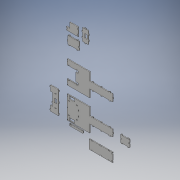
# Autodesk Inventor part: Radio Dowser
Saved by Autodesk Inventor 2018 (Build 220112000, 112)
## iProperties
Created: 2019-04-05
Part Number: Radio Dowser
Material: Generic
Document SubType Name: Modeling
Designer: rpoulter
Density: 1 g/cm^3
Appearance: Default
Author: rpoulter
Autodesk Inventor part; units mm, degrees
ref_plane "YZ Plane" through (0, 0, 0) normal (1, 0, 0) x (0, 1, 0)
ref_plane "XZ Plane" through (0, 0, 0) normal (0, 1, 0) x (-1, 0, 0)
ref_plane "XY Plane" through (0, 0, 0) normal (0, 0, 1) x (1, 0, 0)
sketch "microbit platform" plane through (0, 0, 0) normal (0, 1, 0) x (-1, 0, 0)
  line L0 (0, 0) -> (-46, 0)
  line L1 (-46, 0) -> (-46, -53)
  line L2 (-46, -53) -> (0, -53)
  line L3 (0, -53) -> (0, 0)
  line L4 (-46, -12.5) -> (-43, -12.5)
  line L5 (-43, -12.5) -> (-43, -17.5)
  line L6 (-43, -17.5) -> (-46, -17.5)
  line L7 (-46, -17.5) -> (-46, -12.5)
  line L8 (-46, -35.5) -> (-43, -35.5)
  line L9 (-43, -35.5) -> (-43, -40.5)
  line L10 (-43, -40.5) -> (-46, -40.5)
  line L11 (-46, -40.5) -> (-46, -35.5)
  line L12 (-46, -53) -> (0, -53)
  line L13 (0, -53) -> (0, -45)
  line L14 (0, -45) -> (-46, -45)
  line L15 (-46, -45) -> (-46, -53)
  line L16 (-46, 0) -> (0, 0)
  line L17 (0, 0) -> (0, -8)
  line L18 (0, -8) -> (-46, -8)
  line L19 (-46, -8) -> (-46, 0)
  line L20 (0, 0) -> (-9, 0)
  line L21 (-9, 0) -> (-9, -31)
  line L22 (-9, -31) -> (0, -31)
  line L23 (0, -31) -> (0, 0)
  line L24 (0, -31) -> (6, -31)
  line L25 (6, -31) -> (6, -35.5)
  line L26 (6, -35.5) -> (0, -35.5)
  line L27 (0, -35.5) -> (0, -31)
  line L28 (0, -40.5) -> (6, -40.5)
  line L29 (6, -40.5) -> (6, -45)
  line L30 (6, -45) -> (0, -45)
  line L31 (0, -45) -> (0, -40.5)
  line L32 (0, -40.5) -> (3, -40.5)
  line L33 (3, -40.5) -> (3, -35.5)
  line L34 (3, -35.5) -> (0, -35.5)
  line L35 (0, -35.5) -> (0, -40.5)
  point P0 (0, -35.5)
  dimension "d17" = 46
  dimension "d18" = 53
  dimension "d21" = 3
  dimension "d22" = 5
  dimension "d23" = 5
  dimension "d24" = 8
  dimension "d25" = 8
  dimension "d26" = 9
  dimension "d27" = 31
  dimension "d29" = 4.5
  dimension "d140" = 6
  dimension "d226" = 3
  constraints: 72 end point, 18 parallel, 9 horizontal, 9 perpendicular, 7 point on line, 1 midpoint
  measures "d17" distance of L2.end L1.end
  measures "d18" distance of L1.end L0.end
  measures "d21" distance of L5.end L6.end
  measures "d22" distance of L4.end L5.end
  measures "d23" distance of L8.end L9.end
  measures "d24" distance of L13.end L12.end
  measures "d25" distance of L16.end L17.end
  measures "d26" distance of L22.end L21.end
  measures "d27" distance of L21.end L20.end
  measures "d29" distance between parallel lines of L18 L4
  measures "d140" distance of L25.end L26.end
  measures "d226" distance of L34.end L33.end
extrude "microbit bed" add sketch "microbit platform" along normal blind 3 contours L21 L22 L3 L14 L1 L10 L9 L8 L6 L5 L4 L18 | L24 L25 L26 L3 | L26 L33 L28 L3 | L28 L29 L30 L3
sketch "bed support bottom" plane through (0, 0, 0) normal (0, 1, 0) x (-1, 0, 0)
  line L0 (-46, -8) -> (-46, -12.5) projected
  line L1 (-65.1607, -0.0001) -> (-65.1607, -12.5001)
  line L2 (-46, -12.5) -> (-43, -12.5) projected
  line L3 (-65.1607, -12.5001) -> (-62.1607, -12.5001)
  line L4 (-43, -12.5) -> (-43, -17.5) projected
  line L5 (-62.1607, -12.5001) -> (-62.1607, -17.5001)
  line L6 (-43, -17.5) -> (-46, -17.5) projected
  line L7 (-62.1607, -17.5001) -> (-65.0584, -17.5001)
  line L8 (-46, -17.5) -> (-46, -35.5) projected
  line L9 (-65.0584, -17.5001) -> (-65.0584, -35.5001)
  line L10 (-43, -35.5) -> (-46, -35.5) projected
  line L11 (-65.0584, -35.5001) -> (-62.1607, -35.5001)
  line L12 (-43, -35.5) -> (-43, -40.5) projected
  line L13 (-62.1607, -35.5001) -> (-62.1607, -40.5001)
  line L14 (-43, -40.5) -> (-46, -40.5) projected
  line L15 (-62.1607, -40.5001) -> (-65.0584, -40.5001)
  line L16 (-65.0584, -40.5001) -> (-65.0584, -53.0001)
  line L17 (-90.0584, -53.0001) -> (-90.0584, -40.5001)
  line L18 (-90.0584, -40.5001) -> (-93.0584, -40.5001)
  line L19 (-93.0584, -40.5001) -> (-93.0584, -35.5001)
  line L20 (-93.0584, -35.5001) -> (-90.0584, -35.5001)
  line L21 (-90.0584, -17.5001) -> (-93.0584, -17.5001)
  line L22 (-93.0584, -12.5001) -> (-90.0584, -12.5001)
  line L23 (-90.0584, -17.5001) -> (-90.0584, -35.5001)
  line L24 (-93.0584, -17.5001) -> (-93.0584, -12.5001)
  line L25 (-90.0584, -0.0001) -> (-90.0584, -12.5001)
  line L26 (-80.0584, -0.0001) -> (-80.0584, 2.9999)
  line L27 (-80.0584, 2.9999) -> (-75.0584, 2.9999)
  line L28 (-75.0584, 2.9999) -> (-75.0584, -0.0001)
  line L29 (-80.0584, -53.0001) -> (-80.0584, -56.0001)
  line L30 (-80.0584, -56.0001) -> (-75.0584, -56.0001)
  line L31 (-75.0584, -56.0001) -> (-75.0584, -53.0001)
  line L32 (-65.1607, -0.0001) -> (-75.0584, -0.0001)
  line L33 (-80.0584, -0.0001) -> (-90.0584, -0.0001)
  line L34 (-65.0584, -53.0001) -> (-75.0584, -53.0001)
  line L35 (-80.0584, -53.0001) -> (-90.0584, -53.0001)
  line L36 (-75.0584, -17.5001) -> (-85.0584, -17.5001)
  line L37 (-85.0584, -17.5001) -> (-85.0584, -35.5001)
  line L38 (-85.0584, -35.5001) -> (-75.0584, -35.5001)
  line L39 (-75.0584, -35.5001) -> (-75.0584, -17.5001)
  point P0 (0, 0)
  dimension "d32" = 25
  dimension "d33" = 3
  dimension "d49" = 10
  dimension "d146" = 10
  dimension "d220" = 5
  dimension "d221" = 17.5
  constraints: 64 end point, 14 point on line, 12 parallel, 7 perpendicular, 3 horizontal, 2 vertical
  measures "d32" distance of L16.end L17.start
  measures "d33" distance of L17.end L18.end
  measures "d49" distance between parallel lines of L25 L26
  measures "d146" distance between parallel lines of L37 L39
  measures "d220" distance between parallel lines of L23 L37
  measures "d221" distance between parallel lines of L35 L38
sketch "bed support side x2" plane through (0, 0, 0) normal (0, 1, 0) x (-1, 0, 0)
  line L0 (-46.5564, -81.0331) -> (-43.5564, -81.0331)
  line L1 (-43.5564, -81.0331) -> (-43.5564, -86.0331)
  line L2 (-43.5564, -86.0331) -> (-46.5564, -86.0331)
  line L3 (-8.5564, -96.0331) -> (-8.5564, -99.0331)
  line L4 (-8.5564, -99.0331) -> (-3.5564, -99.0331)
  line L5 (-3.5564, -99.0331) -> (-3.5564, -96.0331)
  line L6 (-38.5564, -96.0331) -> (-38.5564, -99.0331)
  line L7 (-38.5564, -99.0331) -> (-43.5564, -99.0331)
  line L8 (-43.5564, -99.0331) -> (-43.5564, -96.0331)
  line L9 (-46.5564, -71.0331) -> (-46.5564, -62.0331)
  line L10 (-0.5564, -62.0331) -> (-0.5564, -71.0331)
  line L11 (-8.5564, -62.0331) -> (-8.5564, -59.0331)
  line L12 (-8.5564, -59.0331) -> (-3.5564, -59.0331)
  line L13 (-3.5564, -59.0331) -> (-3.5564, -62.0331)
  line L14 (-38.5564, -62.0331) -> (-38.5564, -59.0331)
  line L15 (-38.5564, -59.0331) -> (-43.5564, -59.0331)
  line L16 (-43.5564, -59.0331) -> (-43.5564, -62.0331)
  line L17 (-3.5564, -62.0331) -> (-0.5564, -62.0331)
  line L18 (-46.5564, -62.0331) -> (-43.5564, -62.0331)
  line L19 (-38.5564, -62.0331) -> (-8.5564, -62.0331)
  line L20 (-3.5564, -96.0331) -> (-0.5564, -96.0331)
  line L21 (-46.5564, -96.0331) -> (-43.5564, -96.0331)
  line L22 (-38.5564, -96.0331) -> (-8.5564, -96.0331)
  line L23 (-46.5564, -71.0331) -> (-46.5564, -81.0331)
  line L24 (-46.5564, -86.0331) -> (-46.5564, -96.0331)
  line L25 (-0.5564, -96.0331) -> (-0.5564, -86.0331)
  line L26 (-0.5564, -81.0331) -> (-0.5564, -71.0331)
  line L27 (-0.5564, -81.0331) -> (2.4436, -81.0331)
  line L28 (2.4436, -81.0331) -> (2.4436, -86.0331)
  line L29 (2.4436, -86.0331) -> (-0.5564, -86.0331)
  line L30 (-46.5564, -96.0331) -> (-49.5564, -96.0331)
  line L31 (-49.5564, -96.0331) -> (-49.5564, -86.0331)
  line L32 (-49.5564, -86.0331) -> (-46.5564, -86.0331)
  line L33 (-46.5564, -81.0331) -> (-49.5564, -81.0331)
  line L34 (-49.5564, -81.0331) -> (-49.5564, -62.0331)
  line L35 (-49.5564, -62.0331) -> (-46.5564, -62.0331)
  line L36 (-46.5564, -86.0331) -> (-46.5564, -81.0331)
  point P0 (0, 0)
  dimension "d227" = 3
  dimension "d228" = 3
  constraints: 74 end point, 11 parallel, 9 perpendicular, 9 point on line, 3 collinear, 3 horizontal
  measures "d227" distance of L21.start L8.end
  measures "d228" distance of L21.start L30.end
sketch "top plate" plane through (0, 0, 0) normal (0, 1, 0) x (-1, 0, 0)
  line L0 (3, -153.8907) -> (-97, -153.8907)
  line L1 (-97, -153.8907) -> (-97, -253.8907)
  line L2 (-97, -253.8907) -> (3, -253.8907)
  line L3 (3, -253.8907) -> (3, -153.8907)
  line L4 (3, -177.3907) -> (-46, -177.3907)
  line L5 (-46, -177.3907) -> (-46, -230.3907)
  line L6 (-46, -230.3907) -> (3, -230.3907)
  line L7 (3, -230.3907) -> (3, -177.3907)
  line L8 (-46, -185.3907) -> (-36, -185.3907)
  line L9 (-36, -185.3907) -> (-36, -222.3907)
  line L10 (-36, -222.3907) -> (-46, -222.3907)
  line L11 (-46, -222.3907) -> (-46, -185.3907)
  line L12 (3, -156.595) -> (0, -156.595)
  line L13 (0, -156.595) -> (0, -161.595)
  line L14 (0, -161.595) -> (3, -161.595)
  line L15 (3, -161.595) -> (3, -156.595)
  line L16 (3, -251.316) -> (0, -251.316)
  line L17 (0, -251.316) -> (0, -246.316)
  line L18 (0, -246.316) -> (3, -246.316)
  line L19 (3, -246.316) -> (3, -251.316)
  line L20 (-43, -177.3907) -> (-38, -177.3907)
  line L21 (-38, -177.3907) -> (-38, -174.3907)
  line L22 (-38, -174.3907) -> (-43, -174.3907)
  line L23 (-43, -174.3907) -> (-43, -177.3907)
  line L24 (-8, -177.3907) -> (-3, -177.3907)
  line L25 (-3, -177.3907) -> (-3, -174.3907)
  line L26 (-3, -174.3907) -> (-8, -174.3907)
  line L27 (-8, -174.3907) -> (-8, -177.3907)
  line L28 (-43, -230.3907) -> (-38, -230.3907)
  line L29 (-38, -230.3907) -> (-38, -233.3907)
  line L30 (-38, -233.3907) -> (-43, -233.3907)
  line L31 (-43, -233.3907) -> (-43, -230.3907)
  line L32 (-3, -230.3907) -> (-8, -230.3907)
  line L33 (-8, -230.3907) -> (-8, -233.3907)
  line L34 (-8, -233.3907) -> (-3, -233.3907)
  line L35 (-3, -233.3907) -> (-3, -230.3907)
  line L36 (-97, -188.8907) -> (-197, -188.8907)
  line L37 (-197, -188.8907) -> (-197, -218.8907)
  line L38 (-197, -218.8907) -> (-97, -218.8907)
  line L39 (-97, -218.8907) -> (-97, -188.8907)
  line L40 (-107, -218.8907) -> (-112, -218.8907)
  line L41 (-112, -218.8907) -> (-112, -221.8907)
  line L42 (-112, -221.8907) -> (-107, -221.8907)
  line L43 (-107, -221.8907) -> (-107, -218.8907)
  line L44 (-107, -188.8907) -> (-112, -188.8907)
  line L45 (-112, -188.8907) -> (-112, -185.8907)
  line L46 (-112, -185.8907) -> (-107, -185.8907)
  line L47 (-107, -185.8907) -> (-107, -188.8907)
  line L48 (-144.5, -218.8907) -> (-149.5, -218.8907)
  line L49 (-149.5, -218.8907) -> (-149.5, -221.8907)
  line L50 (-149.5, -221.8907) -> (-144.5, -221.8907)
  line L51 (-144.5, -221.8907) -> (-144.5, -218.8907)
  line L52 (-144.5, -188.8907) -> (-149.5, -188.8907)
  line L53 (-149.5, -188.8907) -> (-149.5, -185.8907)
  line L54 (-149.5, -185.8907) -> (-144.5, -185.8907)
  line L55 (-144.5, -185.8907) -> (-144.5, -188.8907)
  line L56 (-182, -218.8907) -> (-187, -218.8907)
  line L57 (-187, -218.8907) -> (-187, -221.8907)
  line L58 (-187, -221.8907) -> (-182, -221.8907)
  line L59 (-182, -221.8907) -> (-182, -218.8907)
  line L60 (-182, -188.8907) -> (-187, -188.8907)
  line L61 (-187, -188.8907) -> (-187, -185.8907)
  line L62 (-187, -185.8907) -> (-182, -185.8907)
  line L63 (-182, -185.8907) -> (-182, -188.8907)
  line L64 (-197, -201.3907) -> (-200, -201.3907)
  line L65 (-200, -201.3907) -> (-200, -206.3907)
  line L66 (-200, -206.3907) -> (-197, -206.3907)
  line L67 (-197, -206.3907) -> (-197, -201.3907)
  point P0 (0, 0)
  dimension "d63" = 100
  dimension "d64" = 100
  dimension "d65" = 49
  dimension "d66" = 53
  dimension "d67" = 23.5
  dimension "d68" = 10
  dimension "d69" = 37
  dimension "d70" = 8
  dimension "d71" = 3
  dimension "d72" = 5
  dimension "d73" = 3
  dimension "d74" = 5
  dimension "d75" = 5
  dimension "d76" = 3
  dimension "d77" = 3
  dimension "d78" = 5
  dimension "d79" = 3
  dimension "d80" = 30
  dimension "d81" = 3
  dimension "d162" = 100
  dimension "d163" = 30
  dimension "d164" = 35
  dimension "d165" = 5
  dimension "d166" = 3
  dimension "d167" = 3
  dimension "d168" = 5
  dimension "d169" = 5
  dimension "d170" = 3
  dimension "d171" = 5
  dimension "d172" = 12.5
  dimension "d173" = 10
  dimension "d174" = 10
  dimension "d175" = 47.5
  constraints: 136 end point, 34 parallel, 22 point on line, 17 horizontal, 17 perpendicular, 2 collinear
  measures "d63" distance of L2.end L1.end
  measures "d64" distance of L1.end L0.end
  measures "d65" distance of L6.end L5.end
  measures "d66" distance of L5.end L4.end
  measures "d67" distance between parallel lines of L0 L4
  measures "d68" distance of L9.end L10.end
  measures "d69" distance of L8.end L9.end
  measures "d70" distance between parallel lines of L4 L8
  measures "d71" distance of L14.end L13.end
  measures "d72" distance of L13.end L12.end
  measures "d73" distance of L17.end L18.end
  measures "d74" distance of L16.end L17.end
  measures "d75" distance of L22.end L21.end
  measures "d76" distance of L21.end L20.end
  measures "d77" distance between parallel lines of L5 L23
  measures "d78" distance of L26.end L25.end
  measures "d79" distance of L25.end L24.end
  measures "d80" distance between parallel lines of L27 L21
  measures "d81" distance of L28.end L29.end
  measures "d162" distance of L38.end L37.end
  measures "d163" distance of L37.end L36.end
  measures "d164" distance between parallel lines of L0 L36
  measures "d165" distance of L42.end L41.end
  measures "d166" distance of L41.end L40.end
  measures "d167" distance of L44.end L45.end
  measures "d168" distance of L50.end L49.end
  measures "d169" distance of L58.end L57.end
  measures "d170" distance of L66.end L65.end
  measures "d171" distance of L65.end L64.end
  measures "d172" distance between parallel lines of L36 L64
  measures "d173" distance between parallel lines of L37 L57
  measures "d174" distance between parallel lines of L1 L43
  measures "d175" distance between parallel lines of L37 L49
sketch "bottom plate" plane through (0, 0, 0) normal (0, 1, 0) x (-1, 0, 0)
  line L0 (3, -288.3381) -> (-97, -288.3381)
  line L1 (-97, -288.3381) -> (-97, -388.3381)
  line L2 (-97, -388.3381) -> (3, -388.3381)
  line L3 (3, -388.3381) -> (3, -288.3381)
  line L4 (3, -364.8381) -> (3, -311.8381)
  line L5 (3, -291.0423) -> (0, -291.0423)
  line L6 (0, -291.0423) -> (0, -296.0423)
  line L7 (0, -296.0423) -> (3, -296.0423)
  line L8 (3, -296.0423) -> (3, -291.0423)
  line L9 (3, -385.7634) -> (0, -385.7634)
  line L10 (0, -385.7634) -> (0, -380.7634)
  line L11 (0, -380.7634) -> (3, -380.7634)
  line L12 (3, -380.7634) -> (3, -385.7634)
  line L13 (-43, -311.8381) -> (-38, -311.8381)
  line L14 (-38, -311.8381) -> (-38, -308.8381)
  line L15 (-38, -308.8381) -> (-43, -308.8381)
  line L16 (-43, -308.8381) -> (-43, -311.8381)
  line L17 (-8, -311.8381) -> (-3, -311.8381)
  line L18 (-3, -311.8381) -> (-3, -308.8381)
  line L19 (-3, -308.8381) -> (-8, -308.8381)
  line L20 (-8, -308.8381) -> (-8, -311.8381)
  line L21 (-43, -364.8381) -> (-38, -364.8381)
  line L22 (-38, -364.8381) -> (-38, -367.8381)
  line L23 (-38, -367.8381) -> (-43, -367.8381)
  line L24 (-43, -367.8381) -> (-43, -364.8381)
  line L25 (-3, -364.8381) -> (-8, -364.8381)
  line L26 (-8, -364.8381) -> (-8, -367.8381)
  line L27 (-8, -367.8381) -> (-3, -367.8381)
  line L28 (-3, -367.8381) -> (-3, -364.8381)
  line L29 (-46, -324.3381) -> (-49, -324.3381)
  line L30 (-49, -324.3381) -> (-49, -329.3381)
  line L31 (-49, -329.3381) -> (-46, -329.3381)
  line L32 (-46, -329.3381) -> (-46, -324.3381)
  line L33 (-46, -352.3381) -> (-49, -352.3381)
  line L34 (-49, -352.3381) -> (-49, -347.3381)
  line L35 (-49, -347.3381) -> (-46, -347.3381)
  line L36 (-46, -347.3381) -> (-46, -352.3381)
  line L37 (-7, -373.3381) -> (-29, -373.3381)
  line L38 (-29, -373.3381) -> (-29, -385.3381)
  line L39 (-29, -385.3381) -> (-7, -385.3381)
  line L40 (-7, -385.3381) -> (-7, -373.3381)
  line L41 (-7, -291.3381) -> (-29, -291.3381)
  line L42 (-29, -291.3381) -> (-29, -303.3381)
  line L43 (-29, -303.3381) -> (-7, -303.3381)
  line L44 (-7, -303.3381) -> (-7, -291.3381)
  line L45 (3, -335.8381) -> (0, -335.8381)
  line L46 (0, -335.8381) -> (0, -340.8381)
  line L47 (0, -340.8381) -> (3, -340.8381)
  line L48 (3, -340.8381) -> (3, -335.8381)
  line L49 (-97, -323.3381) -> (-197, -323.3381)
  line L50 (-197, -323.3381) -> (-197, -353.3381)
  line L51 (-197, -353.3381) -> (-97, -353.3381)
  line L52 (-97, -353.3381) -> (-97, -323.3381)
  line L53 (-197, -335.8381) -> (-200, -335.8381)
  line L54 (-200, -335.8381) -> (-200, -340.8381)
  line L55 (-200, -340.8381) -> (-197, -340.8381)
  line L56 (-197, -340.8381) -> (-197, -335.8381)
  line L57 (-107, -323.3381) -> (-112, -323.3381)
  line L58 (-112, -323.3381) -> (-112, -320.3381)
  line L59 (-112, -320.3381) -> (-107, -320.3381)
  line L60 (-107, -320.3381) -> (-107, -323.3381)
  line L61 (-187, -323.3381) -> (-182, -323.3381)
  line L62 (-182, -323.3381) -> (-182, -320.3381)
  line L63 (-182, -320.3381) -> (-187, -320.3381)
  line L64 (-187, -320.3381) -> (-187, -323.3381)
  line L65 (-144.5, -323.3381) -> (-149.5, -323.3381)
  line L66 (-149.5, -323.3381) -> (-149.5, -320.3381)
  line L67 (-149.5, -320.3381) -> (-144.5, -320.3381)
  line L68 (-144.5, -320.3381) -> (-144.5, -323.3381)
  line L69 (-107, -353.3381) -> (-112, -353.3381)
  line L70 (-112, -353.3381) -> (-112, -356.3381)
  line L71 (-112, -356.3381) -> (-107, -356.3381)
  line L72 (-107, -356.3381) -> (-107, -353.3381)
  line L73 (-182, -353.3381) -> (-187, -353.3381)
  line L74 (-187, -353.3381) -> (-187, -356.3381)
  line L75 (-187, -356.3381) -> (-182, -356.3381)
  line L76 (-182, -356.3381) -> (-182, -353.3381)
  line L77 (-144.5, -353.3381) -> (-149.5, -353.3381)
  line L78 (-149.5, -353.3381) -> (-149.5, -356.3381)
  line L79 (-149.5, -356.3381) -> (-144.5, -356.3381)
  line L80 (-144.5, -356.3381) -> (-144.5, -353.3381)
  point P0 (0, 0)
  dimension "d82" = 100
  dimension "d83" = 100
  dimension "d90" = 3
  dimension "d91" = 5
  dimension "d92" = 3
  dimension "d93" = 5
  dimension "d94" = 5
  dimension "d95" = 3
  dimension "d97" = 5
  dimension "d98" = 3
  dimension "d99" = 30
  dimension "d100" = 3
  dimension "d101" = 3
  dimension "d102" = 5
  dimension "d103" = 5
  dimension "d104" = 20.5
  dimension "d105" = 12.5
  dimension "d106" = 20.5
  dimension "d108" = 12.5
  dimension "d113" = 22
  dimension "d114" = 12
  dimension "d115" = 3
  dimension "d116" = 10
  dimension "d117" = 22
  dimension "d118" = 12
  dimension "d119" = 5
  dimension "d120" = 47.5
  dimension "d150" = 100
  dimension "d151" = 30
  dimension "d152" = 35
  dimension "d153" = 3
  dimension "d154" = 5
  dimension "d155" = 3
  dimension "d156" = 5
  dimension "d157" = 5
  dimension "d158" = 3
  dimension "d159" = 10
  dimension "d160" = 10
  dimension "d161" = 47.5
  dimension "d213" = 3
  constraints: 162 end point, 40 parallel, 23 point on line, 20 horizontal, 20 perpendicular
  measures "d82" distance of L2.end L2.start
  measures "d83" distance of L2.start L0.end
  measures "d90" distance of L7.end L7.start
  measures "d91" distance of L7.start L5.end
  measures "d92" distance of L10.end L11.end
  measures "d93" distance of L9.end L10.end
  measures "d94" distance of L16.start L14.end
  measures "d95" distance of L14.end L14.start
  measures "d97" distance of L20.start L18.end
  measures "d98" distance of L18.end L18.start
  measures "d99" distance between parallel lines of L20 L14
  measures "d100" distance of L21.end L23.start
  measures "d101" distance of L31.end L30.end
  measures "d102" distance of L30.end L29.end
  measures "d103" distance of L33.end L34.end
  measures "d104" distance between parallel lines of L0 L15
  measures "d105" distance between parallel lines of L13 L29
  measures "d106" distance between parallel lines of L2 L23
  measures "d108" distance between parallel lines of L21 L33
  measures "d113" distance of L39.end L38.end
  measures "d114" distance of L38.end L37.end
  measures "d115" distance between parallel lines of L2 L39
  measures "d116" distance between parallel lines of L3 L40
  measures "d117" distance of L43.end L42.end
  measures "d118" distance of L42.end L41.end
  measures "d119" distance of L46.end L45.end
  measures "d120" distance between parallel lines of L0 L45
  measures "d150" distance of L51.end L50.end
  measures "d151" distance of L50.end L49.end
  measures "d152" distance between parallel lines of L0 L49
  measures "d153" distance of L55.end L54.end
  measures "d154" distance of L58.end L59.end
  measures "d155" distance of L57.end L58.end
  measures "d156" distance of L63.end L62.end
  measures "d157" distance of L66.end L67.end
  measures "d158" distance of L70.end L69.end
  measures "d159" distance between parallel lines of L1 L60
  measures "d160" distance between parallel lines of L50 L64
  measures "d161" distance between parallel lines of L50 L66
  measures "d213" distance between parallel lines of L0 L41
sketch "side support top" plane through (0, 0, 0) normal (0, 1, 0) x (-1, 0, 0)
  line L0 (42.0704, -291.2579) -> (76.0704, -291.2579)
  line L1 (76.0704, -291.2579) -> (76.0704, -391.2579)
  line L2 (76.0704, -391.2579) -> (42.0704, -391.2579)
  line L3 (42.0704, -391.2579) -> (42.0704, -291.2579)
  line L4 (42.0704, -294.2579) -> (39.0704, -294.2579)
  line L5 (39.0704, -294.2579) -> (39.0704, -299.2579)
  line L6 (39.0704, -299.2579) -> (42.0704, -299.2579)
  line L7 (42.0704, -299.2579) -> (42.0704, -294.2579)
  line L8 (42.0704, -388.2579) -> (39.0704, -388.2579)
  line L9 (39.0704, -388.2579) -> (39.0704, -383.2579)
  line L10 (39.0704, -383.2579) -> (42.0704, -383.2579)
  line L11 (42.0704, -383.2579) -> (42.0704, -388.2579)
  line L12 (42.0704, -338.7579) -> (39.0704, -338.7579)
  line L13 (39.0704, -338.7579) -> (39.0704, -343.7579)
  line L14 (39.0704, -343.7579) -> (42.0704, -343.7579)
  line L15 (42.0704, -343.7579) -> (42.0704, -338.7579)
  line L16 (76.0704, -294.2579) -> (79.0704, -294.2579)
  line L17 (79.0704, -294.2579) -> (79.0704, -299.2579)
  line L18 (79.0704, -299.2579) -> (76.0704, -299.2579)
  line L19 (76.0704, -299.2579) -> (76.0704, -294.2579)
  line L20 (76.0704, -388.2579) -> (79.0704, -388.2579)
  line L21 (79.0704, -388.2579) -> (79.0704, -383.2579)
  line L22 (79.0704, -383.2579) -> (76.0704, -383.2579)
  line L23 (76.0704, -383.2579) -> (76.0704, -388.2579)
  line L24 (76.0704, -314.7579) -> (67.0704, -314.7579)
  line L25 (67.0704, -314.7579) -> (67.0704, -367.7579)
  line L26 (67.0704, -367.7579) -> (76.0704, -367.7579)
  line L27 (76.0704, -367.7579) -> (76.0704, -314.7579)
  line L28 (57.0704, -367.7579) -> (52.0704, -367.7579)
  line L29 (52.0704, -367.7579) -> (52.0704, -370.7579)
  line L30 (52.0704, -370.7579) -> (57.0704, -370.7579)
  line L31 (57.0704, -370.7579) -> (57.0704, -367.7579)
  line L32 (57.0704, -314.7579) -> (52.0704, -314.7579)
  line L33 (52.0704, -314.7579) -> (52.0704, -311.7579)
  line L34 (52.0704, -311.7579) -> (57.0704, -311.7579)
  line L35 (57.0704, -311.7579) -> (57.0704, -314.7579)
  line L36 (59.0704, -332.2579) -> (49.0704, -332.2579)
  line L37 (49.0704, -332.2579) -> (49.0704, -350.2579)
  line L38 (49.0704, -350.2579) -> (59.0704, -350.2579)
  line L39 (59.0704, -350.2579) -> (59.0704, -332.2579)
  line L40 (67.0704, -355.2579) -> (70.0704, -355.2579)
  line L41 (70.0704, -355.2579) -> (70.0704, -350.2579)
  line L42 (70.0704, -350.2579) -> (67.0704, -350.2579)
  point P0 (0, 0)
  dimension "d121" = 34
  dimension "d122" = 100
  dimension "d123" = 3
  dimension "d124" = 5
  dimension "d125" = 5
  dimension "d126" = 5
  dimension "d127" = 3
  dimension "d128" = 5
  dimension "d129" = 3
  dimension "d130" = 3
  dimension "d131" = 47.5
  dimension "d132" = 9
  dimension "d133" = 53
  dimension "d134" = 23.5
  dimension "d142" = 5
  dimension "d143" = 3
  dimension "d144" = 10
  dimension "d145" = 3
  dimension "d147" = 10
  dimension "d148" = 18
  dimension "d149" = 41
  dimension "d224" = 3
  dimension "d225" = 5
  constraints: 86 end point, 21 parallel, 14 point on line, 11 horizontal, 11 perpendicular
  measures "d121" distance of L1.end L2.end
  measures "d122" distance of L0.end L1.end
  measures "d123" distance of L6.end L5.end
  measures "d124" distance of L5.end L4.end
  measures "d125" distance of L8.end L9.end
  measures "d126" distance of L13.end L12.end
  measures "d127" distance of L17.end L18.end
  measures "d128" distance of L16.end L17.end
  measures "d129" distance between parallel lines of L0 L4
  measures "d130" distance between parallel lines of L2 L8
  measures "d131" distance between parallel lines of L0 L12
  measures "d132" distance of L26.end L25.end
  measures "d133" distance of L25.end L24.end
  measures "d134" distance between parallel lines of L0 L24
  measures "d142" distance of L30.end L29.end
  measures "d143" distance of L29.end L28.end
  measures "d144" distance between parallel lines of L29 L3
  measures "d145" distance of L32.end L33.end
  measures "d147" distance of L38.end L37.end
  measures "d148" distance of L37.end L36.end
  measures "d149" distance between parallel lines of L0 L36
  measures "d224" distance of L42.end L41.end
  measures "d225" distance of L41.end L40.end
sketch "battery side" plane through (0, 0, 0) normal (0, 1, 0) x (-1, 0, 0)
  line L0 (-94.5331, -411.6252) -> (-197.5331, -411.6252)
  line L1 (-197.5331, -411.6252) -> (-197.5331, -451.6252)
  line L2 (-197.5331, -451.6252) -> (-94.5331, -451.6252)
  line L3 (-94.5331, -451.6252) -> (-94.5331, -411.6252)
  line L4 (-104.5331, -411.6252) -> (-109.5331, -411.6252)
  line L5 (-109.5331, -411.6252) -> (-109.5331, -414.6252)
  line L6 (-109.5331, -414.6252) -> (-104.5331, -414.6252)
  line L7 (-104.5331, -414.6252) -> (-104.5331, -411.6252)
  line L8 (-104.5331, -451.6252) -> (-109.5331, -451.6252)
  line L9 (-109.5331, -451.6252) -> (-109.5331, -448.6252)
  line L10 (-109.5331, -448.6252) -> (-104.5331, -448.6252)
  line L11 (-104.5331, -448.6252) -> (-104.5331, -451.6252)
  line L12 (-142.0331, -411.6252) -> (-147.0331, -411.6252)
  line L13 (-147.0331, -411.6252) -> (-147.0331, -414.6252)
  line L14 (-147.0331, -414.6252) -> (-142.0331, -414.6252)
  line L15 (-142.0331, -414.6252) -> (-142.0331, -411.6252)
  line L16 (-179.5331, -411.6252) -> (-184.5331, -411.6252)
  line L17 (-184.5331, -411.6252) -> (-184.5331, -414.6252)
  line L18 (-184.5331, -414.6252) -> (-179.5331, -414.6252)
  line L19 (-179.5331, -414.6252) -> (-179.5331, -411.6252)
  line L20 (-142.0331, -451.6252) -> (-147.0331, -451.6252)
  line L21 (-147.0331, -451.6252) -> (-147.0331, -448.6252)
  line L22 (-147.0331, -448.6252) -> (-142.0331, -448.6252)
  line L23 (-142.0331, -448.6252) -> (-142.0331, -451.6252)
  line L24 (-179.5331, -451.6252) -> (-184.5331, -451.6252)
  line L25 (-184.5331, -451.6252) -> (-184.5331, -448.6252)
  line L26 (-184.5331, -448.6252) -> (-179.5331, -448.6252)
  line L27 (-179.5331, -448.6252) -> (-179.5331, -451.6252)
  line L28 (-197.5331, -414.6252) -> (-194.5331, -414.6252)
  line L29 (-194.5331, -414.6252) -> (-194.5331, -419.6252)
  line L30 (-194.5331, -419.6252) -> (-197.5331, -419.6252)
  line L31 (-197.5331, -419.6252) -> (-197.5331, -414.6252)
  line L32 (-197.5331, -448.6252) -> (-194.5331, -448.6252)
  line L33 (-194.5331, -448.6252) -> (-194.5331, -443.6252)
  line L34 (-194.5331, -443.6252) -> (-197.5331, -443.6252)
  line L35 (-197.5331, -443.6252) -> (-197.5331, -448.6252)
  point P0 (0, 0)
  dimension "d176" = 103
  dimension "d177" = 40
  dimension "d178" = 5
  dimension "d179" = 3
  dimension "d180" = 3
  dimension "d181" = 5
  dimension "d182" = 5
  dimension "d183" = 5
  dimension "d184" = 10
  dimension "d185" = 13
  dimension "d186" = 50.5
  dimension "d187" = 3
  dimension "d188" = 5
  dimension "d189" = 5
  constraints: 72 end point, 18 parallel, 17 point on line, 9 horizontal, 9 perpendicular, 1 collinear
  measures "d176" distance of L2.end L1.end
  measures "d177" distance of L1.end L0.end
  measures "d178" distance of L6.end L5.end
  measures "d179" distance of L5.end L4.end
  measures "d180" distance of L8.end L9.end
  measures "d181" distance of L14.end L13.end
  measures "d182" distance of L18.end L17.end
  measures "d183" distance of L21.end L22.end
  measures "d184" distance between parallel lines of L3 L7
  measures "d185" distance between parallel lines of L1 L17
  measures "d186" distance between parallel lines of L1 L13
  measures "d187" distance of L29.end L30.end
  measures "d188" distance of L28.end L29.end
  measures "d189" distance of L33.end L32.end
sketch "battery end" plane through (0, 0, 0) normal (0, 1, 0) x (-1, 0, 0)
  line L0 (-232.2978, -326.0929) -> (-272.2978, -326.0929)
  line L1 (-272.2978, -326.0929) -> (-272.2978, -356.0929)
  line L2 (-272.2978, -356.0929) -> (-232.2978, -356.0929)
  line L3 (-232.2978, -356.0929) -> (-232.2978, -326.0929)
  line L4 (-232.2978, -338.5929) -> (-235.2978, -338.5929)
  line L5 (-235.2978, -338.5929) -> (-235.2978, -343.5929)
  line L6 (-235.2978, -343.5929) -> (-232.2978, -343.5929)
  line L7 (-232.2978, -343.5929) -> (-232.2978, -338.5929)
  line L8 (-272.2978, -338.5929) -> (-269.2978, -338.5929)
  line L9 (-269.2978, -338.5929) -> (-269.2978, -342.9302)
  line L10 (-269.2978, -342.9302) -> (-272.2978, -342.9302)
  line L11 (-272.2978, -342.9302) -> (-272.2978, -338.5929)
  line L12 (-235.2978, -326.0929) -> (-240.2978, -326.0929)
  line L13 (-240.2978, -326.0929) -> (-240.2978, -323.0929)
  line L14 (-240.2978, -323.0929) -> (-235.2978, -323.0929)
  line L15 (-235.2978, -323.0929) -> (-235.2978, -326.0929)
  line L16 (-269.2978, -326.0929) -> (-264.2978, -326.0929)
  line L17 (-264.2978, -326.0929) -> (-264.2978, -323.0929)
  line L18 (-264.2978, -323.0929) -> (-269.2978, -323.0929)
  line L19 (-269.2978, -323.0929) -> (-269.2978, -326.0929)
  line L20 (-235.2978, -356.0929) -> (-240.2978, -356.0929)
  line L21 (-240.2978, -356.0929) -> (-240.2978, -359.0929)
  line L22 (-240.2978, -359.0929) -> (-235.2978, -359.0929)
  line L23 (-235.2978, -359.0929) -> (-235.2978, -356.0929)
  line L24 (-264.2978, -356.0929) -> (-269.2978, -356.0929)
  line L25 (-269.2978, -356.0929) -> (-269.2978, -359.0929)
  line L26 (-269.2978, -359.0929) -> (-264.2978, -359.0929)
  line L27 (-264.2978, -359.0929) -> (-264.2978, -356.0929)
  point P0 (0, 0)
  dimension "d190" = 40
  dimension "d191" = 30
  dimension "d192" = 3
  dimension "d193" = 5
  dimension "d194" = 3
  dimension "d195" = 12.5
  dimension "d196" = 12.5
  dimension "d197" = 5
  dimension "d198" = 3
  dimension "d199" = 5
  dimension "d200" = 3
  constraints: 56 end point, 14 parallel, 12 point on line, 7 horizontal, 7 perpendicular
  measures "d190" distance of L2.end L1.end
  measures "d191" distance of L1.end L0.end
  measures "d192" distance of L6.end L5.end
  measures "d193" distance of L5.end L4.end
  measures "d194" distance of L9.end L10.end
  measures "d195" distance between parallel lines of L0 L4
  measures "d196" distance between parallel lines of L0 L8
  measures "d197" distance of L13.end L14.end
  measures "d198" distance of L12.end L13.end
  measures "d199" distance of L18.end L17.end
  measures "d200" distance of L21.end L20.end
extrude "Extrusion2" add sketch "bed support side x2" along normal blind 3
extrude "Extrusion3" add sketch "top plate" along normal blind 3 contours L3 L12 L13 L14 L4 L25 L26 L27 L21 L22 L23 L5 L6 L31 L30 L29 L33 L34 L35 L18 L17 L16 L2 L1 L0 | L1 L38 L37 L36 | L36 L45 L46 L47 | L43 L42 L41 L38 | L36 L53 L54 L55 | L51 L50 L49 L38 | L36 L61 L62 L63 | L59 L58 L57 L38 | L8 L9 L10 L5 | L37 L66 L65 L64
extrude "Extrusion4" add sketch "side support top" along normal blind 3 contours L0 L1 L24 L25 L26 L2 L3 | L3 L6 L5 L4 | L16 L17 L18 L1 | L3 L14 L13 L12 | L3 L8 L9 L10 | L22 L21 L20 L1 | L42 L41 L40 L25
extrude "Extrusion5" add sketch "bottom plate" along normal blind 3 contours L3 L5 L6 L7 L45 L46 L47 L11 L10 L9 L2 L1 L0 | L1 L51 L50 L49 | L49 L58 L59 L60 | L72 L71 L70 L51 | L49 L66 L67 L68 | L80 L79 L78 L51 | L49 L64 L63 L62 | L76 L75 L74 L51 | L50 L55 L54 L53
extrude "Extrusion6" add sketch "battery side" along normal blind 3 contours L3 L2 L11 L10 L9 L23 L22 L21 L27 L26 L25 L1 L32 L33 L34 L30 L29 L28 L0 L17 L18 L19 L13 L14 L15 L5 L6 L7
extrude "Extrusion7" add sketch "battery end" along normal blind 3 contours L3 L4 L5 L6 L2 L1 L10 L9 L8 L0 | L0 L13 L14 L15 | L0 L19 L18 L17 | L23 L22 L21 L2 | L27 L26 L25 L2
sketch "rod" plane through (0, 0, 0) normal (0, 1, 0) x (-1, 0, 0)
  line L0 (-9.5797, -394.9873) -> (-65.5797, -394.9873)
  line L1 (-67.5797, -396.9873) -> (-67.5797, -402.9873)
  line L2 (-65.5797, -404.9873) -> (-9.5797, -404.9873)
  line L3 (-7.5797, -402.9873) -> (-7.5797, -396.9873)
  circle A0 centre (-12.4315, -399.9873) radius 2.3
  arc A1 (-65.5797, -394.9873) -> (-67.5797, -396.9873) centre (-65.5797, -396.9873) ccw
  arc A2 (-67.5797, -402.9873) -> (-65.5797, -404.9873) centre (-65.5797, -402.9873) ccw
  arc A3 (-7.5797, -396.9873) -> (-9.5797, -394.9873) centre (-9.5797, -396.9873) ccw
  arc A4 (-9.5797, -404.9873) -> (-7.5797, -402.9873) centre (-9.5797, -402.9873) ccw
  point P0 (0, 0)
  point P1 (-67.5797, -404.9873)
  point P2 (-67.5797, -394.9873)
  point P3 (-7.5797, -404.9873)
  dimension "d214" = 60
  dimension "d215" = 10
  dimension "d216" = 4.6
  dimension "d217" = 2
  constraints: 8 end point, 8 point on circle, 8 tangent, 6 point on line, 5 centre point, 3 equal radius, 2 parallel, 1 horizontal, 1 perpendicular
  measures "d214" distance of point (-7.58, -404.987) point (-67.58, -404.987)
  measures "d215" distance of point (-67.58, -404.987) point (-67.58, -394.987)
  measures "d216" diameter of A0
  measures "d217" radius of A1
extrude "Extrusion8" add sketch "rod" along normal blind 3
extrude "Extrusion9" add sketch "bed support bottom" along normal blind 3
body "Solid1"
